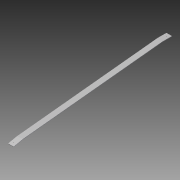
# Autodesk Inventor part: 2p6fs1
Saved by Autodesk Inventor 2014 (Build 180170000, 170)
## iProperties
Company: HERA Project
Created: 2013-12-11
Part Number: 2p6fs1
Material: Steel
Document SubType Name: Sheet Metal
Designer: David DeBoer
Mass: 925.881 g
Surface Area: 993.091 cm^2
Volume: 117.947 cm^3
Density: 7.85 g/cm^3
Description: inner furring strip
Appearance: Steel
Sheet Metal Rule: Default
Author: David DeBoer
Autodesk Inventor part; units mm, degrees
ref_plane "YZ Plane" through (0, 0, 0) normal (1, 0, 0) x (0, 1, 0)
ref_plane "XZ Plane" through (0, 0, 0) normal (0, 1, 0) x (-1, 0, 0)
ref_plane "XY Plane" through (0, 0, 0) normal (0, 0, 1) x (1, 0, 0)
sketch "Sketch1" plane through (0, 0, 0) normal (0, 0, 1) x (1, 0, 0)
  line L0 (0, 0) -> (38.1, 0)
  line L1 (38.1, 0) -> (38.1, 3.048)
  line L2 (38.1, 3.048) -> (0, 3.048)
  line L3 (0, 3.048) -> (0, 0)
  dimension "d0" = 38.1
  dimension "d1" = 3.048
  constraints: 8 end point, 2 parallel, 1 horizontal, 1 perpendicular
  measures "d0" distance of L0.start L0.end
  measures "d1" distance of L2.end L0.start
extrude "Extrusion1" add sketch "Sketch1" along normal blind 1100
sketch "Sketch2" plane through (0, 3.048, 0) normal (0, 1, 0) x (1, 0, 0)
  line L0 (38.1, 0) -> (0, 0) projected
  circle A0 centre (19.05, -20) radius 2.2451
  dimension "d4" = 20
  constraints: 1 centre point
  measures "d4" distance from line of A0.centre L0
hole "Hole1" at (19.05, 3.048, 20) direction (0, -1, 0) diameter 3.175 end through all
sketch "Sketch3" plane through (0, 3.048, 0) normal (0, 1, 0) x (1, 0, 0)
  line L0 (38.1, -1100) -> (0, -1100) projected
  circle A0 centre (19.05, -1080) radius 2.2451
  dimension "d12" = 20
  constraints: 1 centre point
  measures "d12" distance from line of L0 A0.centre
hole "Hole2" at (19.05, 3.048, 1080) direction (0, -1, 0) diameter 3.175 end through all
sketch "Sketch6" plane through (0, 0, 0) normal (0, -1, 0) x (1, 0, 0)
  circle A0 centre (19.05, 20) radius 1.5875 projected
  line L0 (38.1, 0) -> (38.1, 1100) projected
  line L1 (0, 0) -> (0, 1100) projected
  line L2 (0, 60) -> (38.1, 60) construction
  line L3 (0, 60) -> (38.1, 65.016)
  line L4 (0, 60) -> (60.428, 60) construction
  dimension "d29" = 40
  dimension "d30" = 7.5
  constraints: 6 end point, 3 point on line, 1 horizontal, 1 perpendicular
  measures "d29" distance from line of L2 A0.centre
  measures "d30" angle of L4 L3
fold "Fold2" angle 6 bend radius 3.048 thickness 3.048 k factor 0.44 line from (0, 0, 60) to (38.1, 0, 65.016) line at bend centre moving side (-0.1305262, 0, 0.9914449) folds toward (0, -1, 0)
sketch "Sketch7" plane through (0.0184, -0.0167, 60.092) normal (0.0136437, -0.9945219, -0.1036342) x (0.9999067, 0.0136437, 0.0007089)
  line L0 (38.1, 5.016) -> (38.1, 1039.7682) projected
  line L1 (0, 0) -> (0, 1039.7682) projected
  line L2 (0, 977.6655) -> (38.1, 977.6655) construction
  line L3 (0, 977.6655) -> (38.1, 972.6495)
  line L4 (0, 977.6655) -> (38.1, 977.6655) construction
  point P0 (-0.0608, -59.7701)
  dimension "d37" = 7.5
  constraints: 6 end point, 3 point on line, 1 horizontal, 1 perpendicular
  measures "d37" angle of L3 L4
fold "Fold3" angle 6 bend radius 3.048 thickness 3.048 k factor 0.44 line from (0.7115, -101.3363, 1032.4929) to (38.8044, -100.2966, 1027.531) line at bend centre moving side (0.1312169, -0.1009667, 0.9861987) folds toward (0.0136437, -0.9945219, -0.1036342)
equation "\"d1\" = Thickness"
equation "\"d31\" = BendReliefWidth"
equation "\"d32\" = BendReliefDepth"
equation "\"d33\" = MinimumRemnant"
equation "\"d34\" = BendRadius"
equation "\"d36\" = BendRadius"
equation "\"d38\" = BendReliefWidth"
equation "\"d39\" = BendReliefDepth"
equation "\"d40\" = MinimumRemnant"
equation "\"d41\" = BendRadius"
equation "\"d43\" = BendRadius"
equation "\"BendRadius\" = Thickness"
equation "\"BendReliefWidth\" = Thickness"
equation "\"BendReliefDepth\" = 0.5 * Thickness"
equation "\"CornerReliefSize\" = 4 * Thickness"
equation "\"MinimumRemnant\" = 2 * Thickness"
equation "\"TransitionRadius\" = BendRadius"
equation "\"JacobiRadiusSize\" = Thickness"
equation "\"GapSize\" = Thickness"
equation "\"Thickness\" = 3.048"
body "Solid1"
